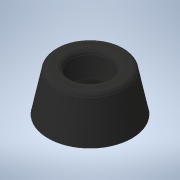
# Autodesk Inventor part: 00-05-001-Rubber
Saved by Autodesk Inventor 2022 (Build 260153000, 153)
## iProperties
Created: 2019-05-31
Part Number: 00-05-001-Rubber
Material: Gummi, Schwarz
Document SubType Name: Modeling
Designer: denni
Density: 0.93 g/cm^3
Appearance: Gummi - Schwarz
Author: denni
Autodesk Inventor part; units mm, degrees
ref_plane "YZ Plane" through (0, 0, 0) normal (1, 0, 0) x (0, 1, 0)
ref_plane "XZ Plane" through (0, 0, 0) normal (0, 1, 0) x (-1, 0, 0)
ref_plane "XY Plane" through (0, 0, 0) normal (0, 0, 1) x (1, 0, 0)
sketch "Skizze1" plane through (0, 0, 0) normal (0, 1, 0) x (-1, 0, 0)
  line L0 (0, 0) -> (0, 10) construction
  line L1 (0, 0) -> (10, 0) construction
  line L2 (10, 0) -> (8, 10) construction
  line L3 (8, 10) -> (0, 10) construction
  line L4 (2.65, 0) -> (10, 0)
  line L5 (10, 0) -> (8, 10)
  line L6 (4.65, 4) -> (7.5, 4)
  line L7 (7.5, 4) -> (7.5, 2.16)
  line L8 (7.5, 2.16) -> (2.65, 2.16)
  line L9 (2.65, 2.16) -> (2.65, 0)
  line L10 (8, 10) -> (4.65, 10)
  line L11 (4.65, 10) -> (4.65, 4)
  dimension "d0" = 16
  dimension "d1" = 20
  dimension "d2" = 10
  dimension "d3" = 9.3
  dimension "d4" = 5.3
  dimension "d5" = 2.16
  dimension "d6" = 6
  dimension "d7" = 15
  constraints: 25 end point, 5 perpendicular, 2 horizontal, 2 point on line, 1 collinear, 1 vertical
  measures "d0" diameter of L2.end L0
  measures "d1" diameter of L1.end L0
  measures "d2" distance between parallel lines of L1 L3
  measures "d3" diameter of L11 L0
  measures "d4" diameter of L9 L0
  measures "d5" distance of L8.end L4.start
  measures "d6" distance of L10.end L6.start
  measures "d7" diameter of L7 L0
revolve "Umdrehung1" add sketch "Skizze1" angle 360 about axis through (0, 0, 0) along (0, 0, 1)
fillet "Rundung1" radius 1 2 edges at (4.65, 0, 10) (8, 0, 10)
